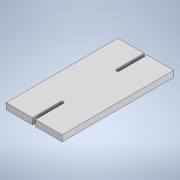
# Autodesk Inventor part: Pièce3
Saved by Autodesk Inventor 2020 (Build 240168000, 168)
## iProperties
Created: 2019-11-07
Part Number: Pièce3
Material: Générique
Document SubType Name: Modeling
Designer: change_le_nom
Density: 1 g/cm^3
Appearance: Par défaut
Author: change_le_nom
Autodesk Inventor part; units mm, degrees
ref_plane "YZ Plane" through (0, 0, 0) normal (1, 0, 0) x (0, 1, 0)
ref_plane "XZ Plane" through (0, 0, 0) normal (0, 1, 0) x (-1, 0, 0)
ref_plane "XY Plane" through (0, 0, 0) normal (0, 0, 1) x (1, 0, 0)
sketch "Esquisse1" plane through (0, 0, 0) normal (0, 1, 0) x (-1, 0, 0)
  line L0 (0, 0) -> (200, 0)
  line L1 (200, 0) -> (200, -400)
  line L2 (200, -400) -> (0, -400)
  line L3 (0, -400) -> (0, 0)
  line L4 (200, -400) -> (200, -313.9237)
  line L5 (100, -400) -> (105, -400)
  line L6 (105, -400) -> (95, -400)
  line L7 (95, -300) -> (95, -400)
  line L8 (95, -400) -> (105, -400)
  line L9 (105, -400) -> (105, -300)
  arc A0 (105, -300) -> (95, -300) centre (100, -300) ccw
  line L10 (105, 0) -> (95, 0)
  line L11 (95, 0) -> (95, -100)
  line L12 (105, -100) -> (105, 0)
  arc A1 (95, -100) -> (105, -100) centre (100, -100) ccw
  dimension "d0" = 200
  dimension "d1" = 400
  dimension "d7" = 100
  constraints: 26 end point, 4 parallel, 4 point on circle, 4 point on line, 2 centre point, 2 horizontal, 2 perpendicular, 1 midpoint
  measures "d0" distance of L1.end L2.end
  measures "d1" distance of L0.end L1.end
  measures "d7" distance of L11.end L10.end
extrude "Extrusion1" add sketch "Esquisse1" along normal blind 22 contours L0 L11 A1 L12 L1 L2 L9 A0 L7 L3
